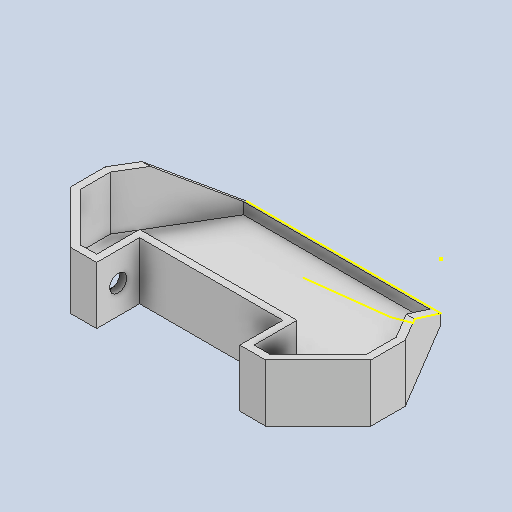
# Autodesk Inventor part: корпус
Saved by Autodesk Inventor 2025 (Build 290162000, 162)
## iProperties
Created: 2025-12-24
Part Number: корпус
Material: Типовые
Document SubType Name: Modeling
Designer: Artem Sannikov
Density: 1 g/cm^3
Appearance: По умолчанию
Author: Artem Sannikov
Autodesk Inventor part; units mm, degrees
ref_plane "YZ Plane" through (0, 0, 0) normal (1, 0, 0) x (0, 1, 0)
ref_plane "XZ Plane" through (0, 0, 0) normal (0, 1, 0) x (-1, 0, 0)
ref_plane "XY Plane" through (0, 0, 0) normal (0, 0, 1) x (1, 0, 0)
sketch "Эскиз1" plane through (0, 0, 0) normal (0, 1, 0) x (-1, 0, 0)
  line L0 (0, 0) -> (-92.3067, 154.5298)
  line L1 (-92.3067, 154.5298) -> (-92.3067, 214.5298)
  line L2 (-92.3067, 214.5298) -> (-0.3828, 306.4537)
  line L3 (-0.3828, 306.4537) -> (44.6172, 306.4537)
  line L4 (44.6172, 306.4537) -> (44.6172, 231.4537)
  line L5 (44.6172, 231.4537) -> (294.6172, 231.4537)
  line L6 (294.6172, 231.4537) -> (294.6172, 306.4537)
  line L7 (294.6172, 306.4537) -> (339.6172, 306.4537)
  line L8 (339.6172, 306.4537) -> (431.5411, 214.5298)
  line L9 (431.5411, 214.5298) -> (431.5411, 154.5298)
  line L10 (431.5411, 154.5298) -> (339.2344, 0)
  line L11 (339.2344, 0) -> (-0.7656, 0)
  point P0 (-92.3067, 184.5298)
  point P1 (431.5411, 184.5298)
  point P2 (-46.1534, 77.2649)
  point P3 (385.3877, 77.2649)
  point P4 (-46.3448, 260.4918)
  point P5 (385.5791, 260.4918)
  point P6 (294.6172, 268.9537)
  point P7 (44.6172, 268.9537)
  dimension "d0" = 180
  dimension "d1" = 130
  dimension "d2" = 45
  dimension "d3" = 75
  dimension "d4" = 60
  dimension "d5" = 180
  dimension "d6" = 250
  dimension "d7" = 340
  constraints: 24 end point, 8 midpoint, 5 perpendicular, 4 equal length, 4 horizontal alignment, 2 parallel, 2 point on line, 1 vertical
  measures "d0" distance of L9.end L10.end
  measures "d1" distance of L7.end L8.end
  measures "d2" distance of L6.end L7.end
  measures "d3" distance of L5.end L6.end
  measures "d4" distance of L0.end L1.end
  measures "d5" distance of L0.start L0.end
  measures "d6" distance of L4.end L5.end
  measures "d7" distance of L10.end L11.end
extrude "Выдавливание1" add sketch "Эскиз1" along normal blind 100
sketch "Эскиз2" plane through (0, 100, 0) normal (0, 1, 0) x (1, 0, 0)
  point P0 (0, 0)
sketch "Эскиз3" plane through (92.3067, 0, 214.5298) normal (1, 0, 0) x (0, 0, -1)
  line L0 (33.7152, 148.0469) -> (238.2174, 0)
  line L1 (238.2174, 0) -> (332.909, 130.8007)
  line L2 (332.909, 130.8007) -> (135.9663, 223.0574)
  line L3 (135.9663, 223.0574) -> (33.7152, 148.0469)
  point P0 (214.5298, 0)
  constraints: 8 end point, 1 perpendicular
extrude "Выдавливание2" cut sketch "Эскиз3" against normal blind 600.5
sketch "Эскиз4" plane through (-407.5973, 100, 114.4458) normal (0, 0.81, -0.5864) x (1, 0, 0)
  line L0 (68.363, 141.2878) -> (407.5973, 141.2878) projected
  line L1 (407.5973, 141.2878) -> (475.9603, 0) projected
  line L2 (499.904, -32.4688) -> (475.9603, 0) projected
  line L3 (499.904, -81.0699) -> (499.904, -32.4688) projected
  line L4 (407.9801, -155.53) -> (499.904, -81.0699) projected
sketch "Эскиз5" plane through (0, 100, 0) normal (0, 1, 0) x (1, 0, 0)
  line L0 (-431.5411, -214.5298) -> (-339.6172, -306.4537) projected
  line L1 (-339.6172, -306.4537) -> (-294.6172, -306.4537) projected
  line L2 (-431.5411, -154.5298) -> (-431.5411, -214.5298) projected
  line L3 (-407.5973, -114.4458) -> (-431.5411, -154.5298) projected
  line L4 (-407.5973, -114.4458) -> (-339.2344, 0) projected
  line L5 (-339.2344, 0) -> (0, 0) projected
  line L6 (0, 0) -> (68.363, -114.4458) projected
  line L7 (92.3067, -154.5298) -> (68.363, -114.4458) projected
  line L8 (92.3067, -214.5298) -> (92.3067, -154.5298) projected
  line L9 (0.3828, -306.4537) -> (92.3067, -214.5298) projected
  line L10 (-44.6172, -306.4537) -> (0.3828, -306.4537) projected
  line L11 (-44.6172, -231.4537) -> (-44.6172, -306.4537) projected
  line L12 (-294.6172, -231.4537) -> (-44.6172, -231.4537) projected
  line L13 (-294.6172, -306.4537) -> (-294.6172, -231.4537) projected
  line L14 (0, -12.3836) -> (-332.2068, -12.3836)
  line L15 (-332.2068, -12.3836) -> (-396.966, -120.7964)
  line L16 (-396.966, -120.7964) -> (-419.1574, -157.9469)
  line L17 (-419.1574, -157.9469) -> (-419.1574, -209.4004)
  line L18 (-419.1574, -209.4004) -> (-334.4877, -294.0701)
  line L19 (-334.4877, -294.0701) -> (-307.0008, -294.0701)
  line L20 (-307.0008, -294.0701) -> (-307.0008, -219.0701)
  line L21 (-307.0008, -219.0701) -> (-32.2335, -219.0701)
  line L22 (-32.2335, -219.0701) -> (-32.2335, -294.0701)
  line L23 (-32.2335, -294.0701) -> (-4.7467, -294.0701)
  line L24 (-4.7467, -294.0701) -> (79.9231, -209.4004)
  line L25 (79.9231, -209.4004) -> (79.9231, -157.9469)
  line L26 (79.9231, -157.9469) -> (57.7316, -120.7964)
  line L27 (57.7316, -120.7964) -> (-10.6313, -6.3505)
  point P0 (-7.0275, -12.3836)
  constraints: 28 end point, 13 other
extrude "Выдавливание3" cut sketch "Эскиз5" against normal blind 93.75 contours L27 L26 L25 L24 L23 L22 L21 L20 L19 L18 L17 L16 L15 L14
sketch "Эскиз6" plane through (0, 6.25, 0) normal (0, 1, 0) x (1, 0, 0)
  line L0 (0, -241.7021) -> (50, -241.7021)
  line L1 (50, -241.7021) -> (50, -126.7021)
  line L2 (50, -126.7021) -> (0, -126.7021)
  line L3 (0, -126.7021) -> (0, -241.7021)
  line L4 (-334.4877, -294.0701) -> (-419.1574, -209.4004) projected
  line L5 (-386.9759, -241.5819) -> (-336.9759, -241.5819)
  line L6 (-336.9759, -241.5819) -> (-336.9759, -126.5819)
  line L7 (-336.9759, -126.5819) -> (-386.9759, -126.5819)
  line L8 (-386.9759, -126.5819) -> (-386.9759, -241.5819)
  point P0 (0, 0)
  point P1 (50, -184.2021)
  point P2 (0, -184.2021)
  point P3 (-336.9759, -184.0819)
  point P4 (-386.9759, -184.0819)
  point P5 (-361.9759, -241.5819)
  point P6 (-361.9759, -126.5819)
  point P7 (25, -241.7021)
  point P8 (25, -126.7021)
  dimension "d23" = 50
  dimension "d24" = 50
  dimension "d25" = 115
  dimension "d26" = 115
  dimension "d27" = 336.9759
  constraints: 16 end point, 8 midpoint, 4 parallel, 2 horizontal, 2 perpendicular, 1 point on line
  measures "d23" distance of point (50, -184.202) point (0, -184.202)
  measures "d24" distance of point (-336.976, -184.082) point (-386.976, -184.082)
  measures "d25" distance of point (-361.976, -241.582) point (-361.976, -126.582)
  measures "d26" distance of point (25, -241.702) point (25, -126.702)
  measures "d27" distance of point (0, -184.202) point (-336.976, -184.082)
extrude "Выдавливание4" cut sketch "Эскиз6" against normal blind 93.75
sketch "Эскиз7" plane through (-294.6172, 0, 306.4537) normal (1, 0, 0) x (0, 0, -1)
  line L0 (0, 100) -> (75, 100) projected
  line L1 (37.5, 100) -> (37.5, 0)
  line L2 (0, 0) -> (75, 0) projected
  line L3 (75, 0) -> (75, 100) projected
  line L4 (75, 50) -> (0, 50)
  line L5 (0, 0) -> (0, 100) projected
  circle A0 centre (37.5, 50) radius 15
  line L6 (-95.282, 50) -> (-21.0844, 50)
  line L7 (-58.1832, 95.9679) -> (-58.1832, 0)
  circle A1 centre (-58.1832, 47.9839) radius 15
  point P0 (306.4537, 0)
  dimension "d30" = 30
  dimension "d31" = 30
  constraints: 8 end point, 6 midpoint, 2 centre point, 1 horizontal, 1 vertical
  measures "d30" diameter of A0
  measures "d31" diameter of A1
extrude "Выдавливание5" cut sketch "Эскиз7" against normal blind 20 contours A0 L4 L1 | L1 L4 A0 | L4 L1 A0 | L4 A0 L1 | A1 L7 L6 | L6 L7 A1 | L7 A1 L6 | L6 A1 L7
sketch "Эскиз8" plane through (-294.6172, 0, 231.4537) normal (0, 0, 1) x (1, 0, 0)
  point P0 (294.6172, 0)
sketch "Эскиз9" plane through (-44.6172, 0, 231.4537) normal (-1, 0, 0) x (0, 0, 1)
  line L0 (0, 0) -> (75, 0) projected
  line L1 (37.5, 0) -> (37.5, 100)
  line L2 (62.6164, 100) -> (-12.3836, 100) projected
  line L3 (75, 0) -> (75, 100) projected
  line L4 (75, 50) -> (1.0391, 50)
  line L5 (1.0391, 50) -> (0, 50)
  line L6 (0, 0) -> (0, 100) projected
  circle A0 centre (38.0196, 50) radius 15
  point P0 (-231.4537, 0)
  dimension "d34" = 30
  constraints: 6 end point, 4 midpoint, 1 centre point, 1 horizontal, 1 point on line, 1 vertical
  measures "d34" diameter of A0
extrude "Выдавливание6" cut sketch "Эскиз9" against normal blind 20 contours A0 L4 L1 | L1 L4 A0 | L4 A0 L1 | L1 A0 L4
